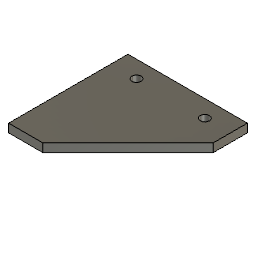
feet_ed (Autodesk Fusion 360 design; units mm, degrees)
Autodesk Fusion 360 part; units mm, degrees
sketch "Sketch1" plane through (0, 0, 0) normal (0, 0, 1) x (1, 0, 0)
  line L0 (-35, 10) -> (35, 10)
  line L1 (35, 10) -> (35, -10)
  line L2 (35, -10) -> (-15, -60)
  line L3 (-15, -60) -> (-35, -60)
  line L4 (-35, -60) -> (-35, 10)
  point P0 (35, 0)
  point P1 (0, 10)
  dimension "d2" = 50
  dimension "d3" = 20
  dimension "d4" = 45
  dimension "d5" = 20
  constraint horizontal L0
  constraint perpendicular L0 L1
  constraint perpendicular L1 L3
  constraint perpendicular L3 L4
  constraint midpoint L1 P0
  constraint midpoint L0 P1
  constraint vertical origin P1
  constraint horizontal origin P0
  measures "d2" vertical distance of L1.end L2.end
  measures "d3" distance of L0.end L1.end
  measures "d4" angle of L2 L3
  measures "d5" distance of L2.end L3.end
extrude "Extrude1" add sketch "Sketch1" along normal blind 5
sketch "Sketch2" plane through (0, 0, 5) normal (0, 0, 1) x (-1, 0, 0)
  line L0 (35, 60) -> (15, 60)
  line L1 (15, 60) -> (-35, 10)
  line L2 (-35, 10) -> (-35, -10)
  line L3 (-35, -10) -> (35, -10)
  line L4 (35, -10) -> (35, 60)
  circle A0 centre (-20, 0) radius 2.7
  circle A1 centre (20, 0) radius 2.7
  dimension "d8" = 5.4
  dimension "d9" = 5.4
  dimension "d10" = 20
  dimension "d11" = 20
  constraint horizontal origin A1.centre
  constraint horizontal origin A0.centre
  measures "d8" diameter of A0
  measures "d9" diameter of A1
  measures "d10" distance of origin A1.centre
  measures "d11" distance of origin A0.centre
extrude "Extrude2" cut sketch "Sketch2" against normal blind 10 contours A0 | A1
